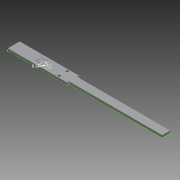
# Autodesk Inventor part: PCB
Saved by Autodesk Inventor 2012 (Build 160160000, 160)
## iProperties
Created: 2014-09-03
Part Number: PCB
Material: Default
Document SubType Name: Modeling
Designer: hannes.maierflaig
Density: 1 g/cm^3
Author: hannes.maierflaig
Autodesk Inventor part; units mm, degrees
ref_plane "YZ Plane" through (0, 0, 0) normal (1, 0, 0) x (0, 1, 0)
ref_plane "XZ Plane" through (0, 0, 0) normal (0, 1, 0) x (-1, 0, 0)
ref_plane "XY Plane" through (0, 0, 0) normal (0, 0, 1) x (1, 0, 0)
sketch "Skizze1" plane through (0, 0, 0) normal (0, 0, 1) x (1, 0, 0)
  line L0 (0, 3) -> (30, 3)
  arc A0 (30, 2.9625) -> (30, 3.0375) centre (30, 3) ccw
  arc A1 (0, 3.0375) -> (0, 2.9625) centre (0, 3) ccw
  line L1 (30, 3) -> (30, 2)
  line L2 (30, 2) -> (77, 2)
  line L3 (77, 2) -> (77, -2)
  line L4 (77, -2) -> (30, -2)
  line L5 (30, -2) -> (30, -3)
  line L6 (0, -3) -> (0, 3)
  circle A2 centre (25, -2) radius 0.6
  line L7 (30, -3) -> (0, -3)
  arc A3 (0, -3.0325) -> (0, -2.9675) centre (0, -3) ccw
  arc A4 (0, 2.9675) -> (0, 3.0325) centre (0, 3) ccw
  arc A5 (-0.0325, 3) -> (0.0325, 3) centre (0, 3) ccw
  arc A6 (29.9675, 3) -> (30.0325, 3) centre (30, 3) ccw
  arc A7 (29.9675, 2) -> (30.0325, 2) centre (30, 2) ccw
  arc A8 (76.9675, 2) -> (77.0325, 2) centre (77, 2) ccw
  arc A9 (77, 2.0325) -> (77, 1.9675) centre (77, 2) ccw
  arc A10 (77, -1.9675) -> (77, -2.0325) centre (77, -2) ccw
  arc A11 (30, -1.9675) -> (30, -2.0325) centre (30, -2) ccw
  arc A12 (30, -2.9675) -> (30, -3.0325) centre (30, -3) ccw
  circle A13 centre (25, 2) radius 0.6
  arc A14 (25, 1.6492) -> (25, 2.3508) centre (25, 2) ccw
  arc A15 (25, 2.3508) -> (25, 1.6492) centre (25, 2) ccw
  arc A16 (25, -2.3508) -> (25, -1.6492) centre (25, -2) ccw
  arc A17 (25, -1.6492) -> (25, -2.3508) centre (25, -2) ccw
  arc A18 (25, 1.6492) -> (25, 2.3508) centre (25, 2) ccw
  arc A19 (25, 2.3508) -> (25, 1.6492) centre (25, 2) ccw
  arc A20 (25, -2.3508) -> (25, -1.6492) centre (25, -2) ccw
  arc A21 (25, -1.6492) -> (25, -2.3508) centre (25, -2) ccw
  circle A22 centre (12.7, 1.27) radius 0.3
  circle A23 centre (12.7, 0) radius 0.3
  circle A24 centre (12.7, -1.27) radius 0.3
  circle A25 centre (13.97, 1.27) radius 0.3
  circle A26 centre (13.97, -1.27) radius 0.3
  arc A27 (35.0325, 0) -> (34.9675, 0) centre (35, 0) ccw
  arc A28 (72.0325, 0) -> (71.9675, 0) centre (72, 0) ccw
  arc A29 (35.0325, 0) -> (34.9675, 0) centre (35, 0) ccw
  arc A30 (30.0325, -2) -> (29.9675, -2) centre (30, -2) ccw
  line L8 (35, 0) -> (72, 0)
  line L9 (12.1968, -0.5032) -> (13.2032, -0.5032)
  line L10 (13.2032, -0.5032) -> (13.2032, 0.5032)
  line L11 (13.2032, 0.5032) -> (12.1968, 0.5032)
  line L12 (12.1968, 0.5032) -> (12.1968, -0.5032)
  line L13 (12.1968, -0.5032) -> (13.2032, -0.5032)
  line L14 (13.2032, -0.5032) -> (13.2032, 0.5032)
  line L15 (13.2032, 0.5032) -> (12.1968, 0.5032)
  line L16 (12.1968, 0.5032) -> (12.1968, -0.5032)
  line L17 (12.0952, -0.6048) -> (13.3048, -0.6048)
  line L18 (13.3048, -0.6048) -> (13.3048, 0.6048)
  line L19 (13.3048, 0.6048) -> (12.0952, 0.6048)
  line L20 (12.0952, 0.6048) -> (12.0952, -0.6048)
  line L21 (12.0952, -0.6048) -> (13.3048, -0.6048)
  line L22 (13.3048, -0.6048) -> (13.3048, 0.6048)
  line L23 (13.3048, 0.6048) -> (12.0952, 0.6048)
  line L24 (12.0952, 0.6048) -> (12.0952, -0.6048)
  line L25 (12.1968, -1.7732) -> (13.2032, -1.7732)
  line L26 (13.2032, -1.7732) -> (13.2032, -0.7668)
  line L27 (13.2032, -0.7668) -> (12.1968, -0.7668)
  line L28 (12.1968, -0.7668) -> (12.1968, -1.7732)
  line L29 (12.1968, -1.7732) -> (13.2032, -1.7732)
  line L30 (13.2032, -1.7732) -> (13.2032, -0.7668)
  line L31 (13.2032, -0.7668) -> (12.1968, -0.7668)
  line L32 (12.1968, -0.7668) -> (12.1968, -1.7732)
  line L33 (12.0952, -1.8748) -> (13.3048, -1.8748)
  line L34 (13.3048, -1.8748) -> (13.3048, -0.6652)
  line L35 (13.3048, -0.6652) -> (12.0952, -0.6652)
  line L36 (12.0952, -0.6652) -> (12.0952, -1.8748)
  line L37 (12.0952, -1.8748) -> (13.3048, -1.8748)
  line L38 (13.3048, -1.8748) -> (13.3048, -0.6652)
  line L39 (13.3048, -0.6652) -> (12.0952, -0.6652)
  line L40 (12.0952, -0.6652) -> (12.0952, -1.8748)
  line L41 (13.4668, 0.7668) -> (14.4732, 0.7668)
  line L42 (14.4732, 0.7668) -> (14.4732, 1.7732)
  line L43 (14.4732, 1.7732) -> (13.4668, 1.7732)
  line L44 (13.4668, 1.7732) -> (13.4668, 0.7668)
  line L45 (13.4668, 0.7668) -> (14.4732, 0.7668)
  line L46 (14.4732, 0.7668) -> (14.4732, 1.7732)
  line L47 (14.4732, 1.7732) -> (13.4668, 1.7732)
  line L48 (13.4668, 1.7732) -> (13.4668, 0.7668)
  line L49 (13.3652, 0.6652) -> (14.5748, 0.6652)
  line L50 (14.5748, 0.6652) -> (14.5748, 1.8748)
  line L51 (14.5748, 1.8748) -> (13.3652, 1.8748)
  line L52 (13.3652, 1.8748) -> (13.3652, 0.6652)
  line L53 (13.3652, 0.6652) -> (14.5748, 0.6652)
  line L54 (14.5748, 0.6652) -> (14.5748, 1.8748)
  line L55 (14.5748, 1.8748) -> (13.3652, 1.8748)
  line L56 (13.3652, 1.8748) -> (13.3652, 0.6652)
  line L57 (13.4668, -1.7732) -> (14.4732, -1.7732)
  line L58 (14.4732, -1.7732) -> (14.4732, -0.7668)
  line L59 (14.4732, -0.7668) -> (13.4668, -0.7668)
  line L60 (13.4668, -0.7668) -> (13.4668, -1.7732)
  line L61 (13.4668, -1.7732) -> (14.4732, -1.7732)
  line L62 (14.4732, -1.7732) -> (14.4732, -0.7668)
  line L63 (14.4732, -0.7668) -> (13.4668, -0.7668)
  line L64 (13.4668, -0.7668) -> (13.4668, -1.7732)
  line L65 (13.3652, -1.8748) -> (14.5748, -1.8748)
  line L66 (14.5748, -1.8748) -> (14.5748, -0.6652)
  line L67 (14.5748, -0.6652) -> (13.3652, -0.6652)
  line L68 (13.3652, -0.6652) -> (13.3652, -1.8748)
  line L69 (13.3652, -1.8748) -> (14.5748, -1.8748)
  line L70 (14.5748, -1.8748) -> (14.5748, -0.6652)
  line L71 (14.5748, -0.6652) -> (13.3652, -0.6652)
  line L72 (13.3652, -0.6652) -> (13.3652, -1.8748)
  line L73 (12.1968, 0.7668) -> (13.2032, 0.7668)
  line L74 (13.2032, 0.7668) -> (13.2032, 1.7732)
  line L75 (13.2032, 1.7732) -> (12.1968, 1.7732)
  line L76 (12.1968, 1.7732) -> (12.1968, 0.7668)
  line L77 (12.1968, 0.7668) -> (13.2032, 0.7668)
  line L78 (13.2032, 0.7668) -> (13.2032, 1.7732)
  line L79 (13.2032, 1.7732) -> (12.1968, 1.7732)
  line L80 (12.1968, 1.7732) -> (12.1968, 0.7668)
  line L81 (12.0952, 0.6652) -> (13.3048, 0.6652)
  line L82 (13.3048, 0.6652) -> (13.3048, 1.8748)
  line L83 (13.3048, 1.8748) -> (12.0952, 1.8748)
  line L84 (12.0952, 1.8748) -> (12.0952, 0.6652)
  line L85 (12.0952, 0.6652) -> (13.3048, 0.6652)
  line L86 (13.3048, 0.6652) -> (13.3048, 1.8748)
  line L87 (13.3048, 1.8748) -> (12.0952, 1.8748)
  line L88 (12.0952, 1.8748) -> (12.0952, 0.6652)
  line L89 (0, 3) -> (30, 3)
  line L90 (30, 3) -> (30, -3)
  line L91 (30, -3) -> (0, -3)
  line L92 (0, -3) -> (0, 3)
  line L93 (30, 2) -> (77, 2)
  line L94 (77, 2) -> (77, -2)
  line L95 (77, -2) -> (30, -2)
  line L96 (30, -2) -> (30, 2)
  line L97 (14.7384, 0.7621) -> (15.7448, 0.7621)
  line L98 (15.7448, 0.7621) -> (15.7448, 1.7685)
  line L99 (15.7448, 1.7685) -> (14.7384, 1.7685)
  line L100 (14.7384, 1.7685) -> (14.7384, 0.7621)
  line L101 (14.7384, 0.7621) -> (15.7448, 0.7621)
  line L102 (15.7448, 0.7621) -> (15.7448, 1.7685)
  line L103 (15.7448, 1.7685) -> (14.7384, 1.7685)
  line L104 (14.6368, 0.6605) -> (15.8464, 0.6605)
  line L105 (15.8464, 0.6605) -> (15.8464, 1.8701)
  line L106 (15.8464, 1.8701) -> (14.6368, 1.8701)
  line L107 (14.6368, 0.6605) -> (15.8464, 0.6605)
  line L108 (15.8464, 0.6605) -> (15.8464, 1.8701)
  line L109 (15.8464, 1.8701) -> (14.6368, 1.8701)
  line L110 (14.6368, 1.8701) -> (14.6368, 0.6605)
  line L111 (14.7384, -1.7779) -> (15.7448, -1.7779)
  line L112 (15.7448, -1.7779) -> (15.7448, -0.7715)
  line L113 (15.7448, -0.7715) -> (14.7384, -0.7715)
  line L114 (14.7384, -1.7779) -> (15.7448, -1.7779)
  line L115 (15.7448, -1.7779) -> (15.7448, -0.7715)
  line L116 (15.7448, -0.7715) -> (14.7384, -0.7715)
  line L117 (14.7384, -0.7715) -> (14.7384, -1.7779)
  line L118 (14.6368, -1.8795) -> (15.8464, -1.8795)
  line L119 (15.8464, -1.8795) -> (15.8464, -0.6699)
  line L120 (15.8464, -0.6699) -> (14.6368, -0.6699)
  line L121 (14.6368, -1.8795) -> (15.8464, -1.8795)
  line L122 (15.8464, -1.8795) -> (15.8464, -0.6699)
  line L123 (15.8464, -0.6699) -> (14.6368, -0.6699)
  line L124 (14.6368, -0.6699) -> (14.6368, -1.8795)
  circle A31 centre (15.24, 1.27) radius 0.3
  circle A32 centre (15.24, -1.2747) radius 0.3
  point P0 (0, 0)
  dimension "d11" = 0.6
  dimension "d12" = 0.6
  dimension "d13" = 0.6
  constraints: 250 end point, 48 point on circle, 33 centre point, 4 parallel, 3 coincident, 2 horizontal, 2 perpendicular
  measures "d11" diameter of A26
  measures "d12" diameter of A31
  measures "d13" diameter of A32
extrude "Extrusion1" add sketch "Skizze1" along normal blind 1 contours L0 A4 L6 | L0 A6 L1 L90 A11 L5 A12 L7 A3 L6 A4 | L0 L1 A6 | A3 L7 L6 | A12 L5 L7 | L90 L5 A11 | L12 L11 L10 L9 | L20 L19 L18 L17 | L28 L27 L26 L25 | L36 L35 L34 L33 | L44 L43 L42 L41 | L52 L51 L50 L49 | L60 L59 L58 L57 | L68 L67 L66 L65 | L76 L75 L74 L73 | L84 L83 L82 L81 | L100 L99 L98 L97 | L110 L106 L105 L104 | L117 L113 L112 L111 | L124 L120 L119 L118 | A31 | A32
extrude "Extrusion4" add sketch "Skizze1" along normal blind 1 contours L2 A7 L90 | L2 A8 L3 A10 L4 A30 L90 A7 | L2 L3 A8 | A30 L4 L90 | L3 L4 A10
extrude "Extrusion5" cut sketch "Skizze1" along normal blind 10 contours A31 | A32
